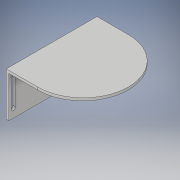
# Autodesk Inventor part: Glas und Flaschenboden
Saved by Autodesk Inventor 2019 (Build 230136000, 136)
## iProperties
Created: 2018-09-20
Part Number: Glas und Flaschenboden
Material: Generisch
Document SubType Name: Modeling
Designer: nico-
Density: 1 g/cm^3
Appearance: Vorgabe
Author: nico-
Autodesk Inventor part; units mm, degrees
ref_plane "YZ Plane" through (0, 0, 0) normal (1, 0, 0) x (0, 1, 0)
ref_plane "XZ Plane" through (0, 0, 0) normal (0, 1, 0) x (-1, 0, 0)
ref_plane "XY Plane" through (0, 0, 0) normal (0, 0, 1) x (1, 0, 0)
sketch "Skizze1" plane through (0, 0, 0) normal (0, 0, 1) x (1, 0, 0)
  line L0 (0, 0) -> (0, -50)
  line L1 (0, 0) -> (50, 0) construction
  line L2 (0, -50) -> (3, -50)
  line L3 (3, -50) -> (3, -3)
  line L4 (3, -3) -> (88, -3)
  line L5 (88, -3) -> (88, 0)
  line L6 (88, 0) -> (0, 0)
  dimension "d0" = 50
  dimension "d1" = 90
  dimension "d2" = 3
  dimension "d3" = 47
  dimension "d4" = 85
  dimension "d5" = 90
  constraints: 14 end point, 6 perpendicular, 1 horizontal, 1 vertical
  measures "d0" distance of L0.start L0.end
  measures "d1" angle of L0 L1
  measures "d2" distance of L0.end L2.end
  measures "d3" distance of L2.end L3.end
  measures "d4" distance of L3.end L4.end
  measures "d5" angle of L3 L4
extrude "Extrusion1" add sketch "Skizze1" along normal mid plane 104
fillet "Rundung1" radius 52 2 edges at (88, -1.5, -52) (88, -1.5, 52)
sketch "Skizze2" plane through (3, -50, 52) normal (1, 0, 0) x (0, 0, -1)
  line L0 (2.5, 40) -> (7.5, 40)
  line L1 (7.5, 40) -> (7.5, 10)
  line L2 (7.5, 10) -> (2.5, 10)
  line L3 (2.5, 10) -> (2.5, 40)
  arc A0 (7.5, 40) -> (2.5, 40) centre (5, 40) ccw
  arc A1 (2.5, 10) -> (7.5, 10) centre (5, 10) ccw
  point P0 (52, 50)
  dimension "d9" = 5
  dimension "d10" = 30
  constraints: 8 end point, 4 point on circle, 2 centre point, 2 midpoint, 2 parallel, 1 horizontal, 1 perpendicular
  measures "d9" distance of L1.end L2.end
  measures "d10" distance of L0.end L1.end
extrude "Extrusion2" cut sketch "Skizze2" against normal blind 3
sketch "Skizze3" plane through (3, -50, 52) normal (1, 0, 0) x (0, 0, -1)
  line L0 (101.5, 40) -> (96.5, 40)
  line L1 (96.5, 40) -> (96.5, 10)
  line L2 (96.5, 10) -> (101.5, 10)
  line L3 (101.5, 10) -> (101.5, 40)
  arc A0 (101.5, 40) -> (96.5, 40) centre (99, 40) ccw
  arc A1 (96.5, 10) -> (101.5, 10) centre (99, 10) ccw
  point P0 (52, 50)
  dimension "d13" = 5
  dimension "d14" = 30
  constraints: 8 end point, 4 point on circle, 2 centre point, 2 midpoint, 2 parallel, 1 horizontal, 1 perpendicular
  measures "d13" distance of L2.end L1.end
  measures "d14" distance of L1.end L0.end
extrude "Extrusion3" cut sketch "Skizze3" against normal blind 3
